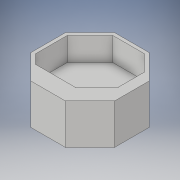
# Autodesk Inventor part: 示範一
Saved by Autodesk Inventor 2017 (Build 210142000, 142)
## iProperties
Part Number: 示範一
Material: 一般
Document SubType Name: Modeling
Designer: user
Density: 1 g/cm^3
Appearance: 預設
Author: user
Autodesk Inventor part; units mm, degrees
ref_plane "YZ Plane" through (0, 0, 0) normal (1, 0, 0) x (0, 1, 0)
ref_plane "XZ Plane" through (0, 0, 0) normal (0, 1, 0) x (-1, 0, 0)
ref_plane "XY Plane" through (0, 0, 0) normal (0, 0, 1) x (1, 0, 0)
sketch "草圖1" plane through (0, 0, 0) normal (0, 1, 0) x (-1, 0, 0)
  line L0 (-12.5, 5.1777) -> (-5.1777, 12.5)
  line L1 (-5.1777, 12.5) -> (5.1777, 12.5)
  line L2 (5.1777, 12.5) -> (12.5, 5.1777)
  line L3 (12.5, 5.1777) -> (12.5, -5.1777)
  line L4 (12.5, -5.1777) -> (5.1777, -12.5)
  line L5 (5.1777, -12.5) -> (-5.1777, -12.5)
  line L6 (-5.1777, -12.5) -> (-12.5, -5.1777)
  line L7 (-12.5, -5.1777) -> (-12.5, 5.1777)
  line L8 (123.9504, 0) -> (-90.7739, 0) construction
  point P0 (0, 0)
  point P1 (0, 0)
  dimension "d1" = 25
  constraints: 18 end point, 1 coincident, 1 horizontal, 1 parallel, 1 point on line, 17 other
  measures "d1" distance between parallel lines of L1 L5
extrude "擠出1" add sketch "草圖1" along normal blind 12
shell "薄殼3" thickness 5 removed faces 1 at (-0.7149, 12, -1.7259) ; own thickness 5 on faces at (1.7259, 4, 12.5) (10.0592, 4, 7.6184) ; own thickness 3 on faces at (12.5, 4, -1.7259) ; own thickness 1 on faces at (-7.6184, 4, 10.0592) (-12.5, 4, 1.7259) (-10.0592, 4, -7.6184) (-1.7259, 4, -12.5) (7.6184, 4, -10.0592)
